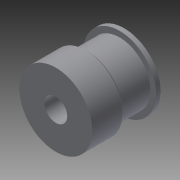
# Autodesk Inventor part: gt2_20_pulley
Saved by Autodesk Inventor 2013 (Build 170138000, 138)
## iProperties
Created: 2014-04-01
Part Number: gt2_20_pulley
Material: Generic
Document SubType Name: Modeling
Designer: dzban
Density: 1 g/cm^3
Author: dzban
Autodesk Inventor part; units mm, degrees
ref_plane "YZ Plane" through (0, 0, 0) normal (1, 0, 0) x (0, 1, 0)
ref_plane "XZ Plane" through (0, 0, 0) normal (0, 1, 0) x (-1, 0, 0)
ref_plane "XY Plane" through (0, 0, 0) normal (0, 0, 1) x (1, 0, 0)
sketch "Sketch1" plane through (0, 0, 0) normal (0, 0, 1) x (1, 0, 0)
  line L0 (0, 0) -> (0, 15)
  line L1 (0, 15) -> (5.5, 15)
  line L2 (5.5, 15) -> (5.5, 14)
  line L3 (5.5, 14) -> (4.25, 14)
  line L4 (4.25, 14) -> (4.25, 7)
  line L5 (4.25, 7) -> (5.1, 7)
  line L6 (5.5, 6.6) -> (5.5, 0)
  line L7 (5.5, 0) -> (0, 0)
  line L8 (-2.5, 11.781) -> (-2.5, 3.2351)
  line L9 (5.5, 6.6) -> (5.1, 7)
  point P0 (5.5, 7)
  dimension "d0" = 5.5
  dimension "d1" = 7
  dimension "d2" = 7
  dimension "d4" = 2.5
  dimension "d6" = 15
  dimension "d7" = 4.25
  dimension "d8" = 0.4
  dimension "d9" = 0.4
  constraints: 20 end point, 4 parallel, 4 perpendicular, 2 point on line, 1 collinear, 1 vertical
  measures "d0" distance between parallel lines of L6 L0
  measures "d1" distance between parallel lines of L5 L7
  measures "d2" distance between parallel lines of L3 L5
  measures "d4" distance between parallel lines of L0 L8
  measures "d6" distance between parallel lines of L1 L7
  measures "d7" distance between parallel lines of L4 L0
  measures "d8" distance of L6.start point (5.5, 7)
  measures "d9" distance of L5.end point (5.5, 7)
revolve "Revolution2" add sketch "Sketch1" angle 360 about axis through (-2.5, 11.781, 0) along (0, -1, 0)
equation "\"d9\" = d8"
body "Solid2"
